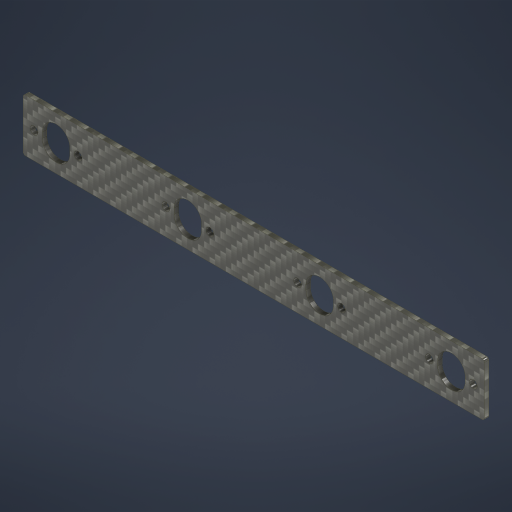
# Autodesk Inventor part: Leg_Loadpipe_Plate
Saved by Autodesk Inventor 2024 (Build 280153000, 153)
## iProperties
Created: 2023-06-08
Part Number: Leg_Loadpipe_Plate
Material: CFRP
Document SubType Name: Modeling
Designer: dzw04
Density: 1.43 g/cm^3
Appearance: Carbon Fiber 1
Author: dzw04
Autodesk Inventor part; units mm, degrees
ref_plane "YZ Plane" through (0, 0, 0) normal (1, 0, 0) x (0, 1, 0)
ref_plane "XZ Plane" through (0, 0, 0) normal (0, 1, 0) x (-1, 0, 0)
ref_plane "XY Plane" through (0, 0, 0) normal (0, 0, 1) x (1, 0, 0)
sketch "Sketch1" plane through (0, 0, 0) normal (0, 0, 1) x (1, 0, 0)
  line L0 (0, -7) -> (208, -7)
  line L1 (209, -8) -> (209, -30)
  line L2 (208, -31) -> (0, -31)
  line L3 (-1, -30) -> (-1, -8)
  circle A0 centre (38.25, -10.75) radius 1.75
  circle A1 centre (58.75, -10.75) radius 1.75
  circle A2 centre (149.25, -10.75) radius 1.75
  circle A3 centre (169.75, -10.75) radius 1.75
  circle A4 centre (38.25, -40.75) radius 1.75
  circle A5 centre (58.75, -40.75) radius 1.75
  circle A6 centre (149.25, -40.75) radius 1.75
  circle A7 centre (169.75, -40.75) radius 1.75
  arc A8 (0, -7) -> (-1, -8) centre (0, -8) ccw
  arc A9 (-1, -30) -> (0, -31) centre (0, -30) ccw
  arc A10 (208, -31) -> (209, -30) centre (208, -30) ccw
  arc A11 (209, -8) -> (208, -7) centre (208, -8) ccw
  point P0 (0, 0)
  point P1 (209, -31)
  point P2 (209, -7)
  point P3 (-1, -31)
  dimension "d0" = 210
  dimension "d1" = 24
  dimension "d10" = 111
  dimension "d13" = 30
  dimension "d16" = 1
  constraints: 12 centre point, 8 end point, 8 point on circle, 8 tangent, 6 point on line, 3 equal radius, 2 horizontal, 2 parallel, 1 perpendicular, 1 vertical, 12 other
  measures "d0" distance of point (209, -31) point (-1, -31)
  measures "d1" distance of point (209, -7) point (209, -31)
  measures "d10" distance of A0.centre A2.centre
  measures "d13" distance of A0.centre A4.centre
  measures "d16" radius of A8
extrude "Extrusion1" add sketch "Sketch1" along normal blind 2 contours L0 A11 L1 A10 L2 A9 L3 A8 | A0 | A1 | A2 | A3
sketch "Sketch2" plane through (0, 0, 2) normal (0, 0, 1) x (1, 0, 0)
  line L0 (209, -30) -> (209, -8) projected
  line L1 (209, -19) -> (-1, -19) construction
  line L2 (-1, -8) -> (-1, -30) projected
  line L3 (235.9536, -47.1551) -> (247.5417, -11.4905)
  line L4 (235.9536, -47.1551) -> (273.4536, -47.1551) construction
  line L5 (235.9536, -47.1551) -> (237.8557, -47.7731)
  line L6 (235.9536, -47.1551) -> (237.9536, -47.1551) construction
  line L7 (237.8557, -47.7731) -> (249.4438, -12.1085)
  line L8 (249.4438, -12.1085) -> (247.5417, -11.4905)
  line L9 (249.4438, -12.1085) -> (271.3181, -19.2159)
  line L10 (271.3181, -19.2159) -> (259.73, -54.8805)
  line L11 (259.73, -54.8805) -> (261.6321, -55.4986)
  line L12 (261.6321, -55.4986) -> (273.2202, -19.8339)
  line L13 (273.2202, -19.8339) -> (271.3181, -19.2159)
  line L14 (265.5241, -37.0482) -> (243.6498, -29.9408)
  line L15 (177.3204, -33.4945) -> (331.8534, -33.4945)
  line L16 (244.4446, -27.4945) -> (242.5425, -26.8765)
  line L17 (238.4427, -39.4945) -> (240.3448, -40.1125)
  line L18 (244.4446, -27.4945) -> (240.3448, -40.1125)
  line L19 (104, -19) -> (104, -19)
  line L20 (104, -19) -> (104, -19) construction
  line L21 (104, -20.25) -> (104, -17.75) construction
  line L22 (110.25, -20.25) -> (110.25, -17.75)
  line L23 (97.75, -17.75) -> (97.75, -20.25)
  arc A0 (97.75, -20.25) -> (110.25, -20.25) centre (104, -20.25) ccw
  arc A1 (110.25, -17.75) -> (97.75, -17.75) centre (104, -17.75) ccw
  line L24 (104, -19) -> (74, -19) construction
  line L25 (104, -19) -> (134, -19) construction
  line L26 (74, -20.25) -> (74, -17.75) construction
  line L27 (80.25, -20.25) -> (80.25, -17.75)
  line L28 (67.75, -17.75) -> (67.75, -20.25)
  arc A2 (67.75, -20.25) -> (80.25, -20.25) centre (74, -20.25) ccw
  arc A3 (80.25, -17.75) -> (67.75, -17.75) centre (74, -17.75) ccw
  line L29 (134, -20) -> (134, -18) construction
  line L30 (140.25, -20) -> (140.25, -18)
  line L31 (127.75, -18) -> (127.75, -20)
  arc A4 (127.75, -20) -> (140.25, -20) centre (134, -20) ccw
  arc A5 (140.25, -18) -> (127.75, -18) centre (134, -18) ccw
  line L32 (74, -19) -> (14, -19) construction
  line L33 (134, -19) -> (194, -19) construction
  line L34 (194, -20) -> (194, -18) construction
  line L35 (200.25, -20) -> (200.25, -18)
  line L36 (187.75, -18) -> (187.75, -20)
  arc A6 (187.75, -20) -> (200.25, -20) centre (194, -20) ccw
  arc A7 (200.25, -18) -> (187.75, -18) centre (194, -18) ccw
  line L37 (14, -20.25) -> (14, -17.75) construction
  line L38 (20.25, -20.25) -> (20.25, -17.75)
  line L39 (7.75, -17.75) -> (7.75, -20.25)
  arc A8 (7.75, -20.25) -> (20.25, -20.25) centre (14, -20.25) ccw
  arc A9 (20.25, -17.75) -> (7.75, -17.75) centre (14, -17.75) ccw
  circle A10 centre (14, -19) radius 10 construction
  line L40 (14, -19) -> (24.6066, -8.3934) construction
  line L41 (14, -19) -> (29, -19) construction
  line L42 (14, -19) -> (3.3934, -29.6066) construction
  circle A11 centre (4, -19) radius 1.75
  circle A12 centre (24, -19) radius 1.75
  circle A13 centre (54, -19) radius 1.75
  circle A14 centre (34, -19) radius 1.75
  circle A15 centre (84, -19) radius 1.75
  circle A16 centre (64, -19) radius 1.75
  circle A17 centre (114, -19) radius 1.75
  circle A18 centre (94, -19) radius 1.75
  circle A19 centre (144, -19) radius 1.75
  circle A20 centre (124, -19) radius 1.75
  circle A21 centre (174, -19) radius 1.75
  circle A22 centre (154, -19) radius 1.75
  circle A23 centre (204, -19) radius 1.75
  circle A24 centre (184, -19) radius 1.75
  point P0 (0, 0)
  point P1 (254.5869, -33.4945)
  dimension "d19" = 37.5
  dimension "d20" = 72
  dimension "d21" = 2
  dimension "d22" = 18
  dimension "d23" = 37.5
  dimension "d24" = 23
  dimension "d25" = 37.5
  dimension "d26" = 90
  dimension "d27" = 2
  dimension "d28" = 37.5
  dimension "d29" = 90
  dimension "d32" = 0
  dimension "d33" = 90
  dimension "d34" = 1.25
  dimension "d35" = 12.5
  dimension "d38" = 30
  dimension "d39" = 30
  dimension "d40" = 1.25
  dimension "d41" = 12.5
  dimension "d42" = 1
  dimension "d43" = 12.5
  dimension "d44" = 60
  dimension "d45" = 60
  dimension "d46" = 1
  dimension "d47" = 12.5
  dimension "d48" = 1.25
  dimension "d49" = 12.5
  dimension "d50" = 20
  dimension "d51" = 15
  dimension "d52" = 45
  dimension "d53" = 15
  dimension "d63" = 3.5
  dimension "d64" = 3.5
  dimension "d67" = 30
  constraints: 92 end point, 25 centre point, 22 point on circle, 20 tangent, 12 midpoint, 9 horizontal, 8 parallel, 6 point on line, 5 perpendicular, 4 equal length, 3 vertical, 1 coincident, 1 collinear, 24 other
  measures "d19" distance of L3.start L3.end
  measures "d20" angle of L4 L3
  measures "d21" distance of L3.start L5.end
  measures "d22" angle of L5 L6
  measures "d23" distance of L5.end L7.end
  measures "d24" distance of L7.end L9.end
  measures "d25" distance of L9.end L10.end
  measures "d26" angle of L9 L10
  measures "d27" distance of L10.end L11.end
  measures "d28" distance of L11.end L12.end
  measures "d29" angle of L12 L11
  measures "d32" distance of L19.start L19.end
  measures "d33" angle of L19 L20
  measures "d34" distance of L19.end L21.end
  measures "d35" diameter of A1
  measures "d38" distance of L19.end L24.end
  measures "d39" distance of L19.end L25.end
  measures "d40" distance of L24.end L26.end
  measures "d41" diameter of A3
  measures "d42" distance of L25.end L29.end
  measures "d43" diameter of A5
  measures "d44" distance of L24.end L32.end
  measures "d45" distance of L25.end L33.end
  measures "d46" distance of L33.end L34.end
  measures "d47" diameter of A7
  measures "d48" distance of L32.end L37.end
  measures "d49" diameter of A9
  measures "d50" diameter of A10
  measures "d51" distance of L40.start L40.end
  measures "d52" angle of L41 L40
  measures "d53" distance of L40.start L42.end
  measures "d63" diameter of A11
  measures "d64" diameter of A12
  measures "d67" distance of A12.centre A13.centre
extrude "Extrusion2" cut sketch "Sketch2" against normal blind 10 contours A2 L28 A3 L27 | A4 L31 A5 L30 | A6 L36 A7 L35 | A8 L39 A9 L38 | A11 | A12 | A15 | A16 | A19 | A20 | A23 | A24
body "Solid1"
